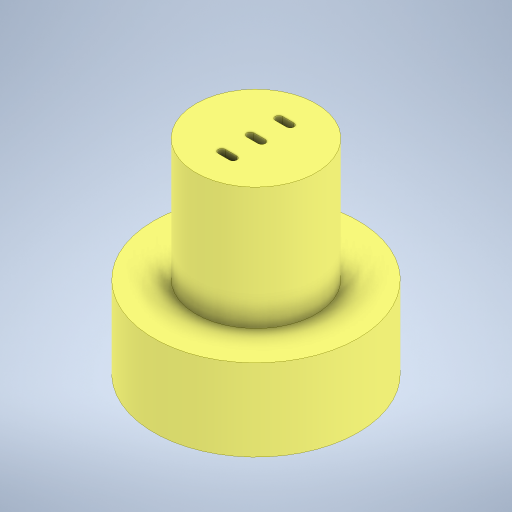
# Autodesk Inventor part: Kabelstopfen_Hinten_next try
Saved by Autodesk Inventor 2023 (Build 270158030, 158C)
## iProperties
Created: 2020-02-25
Part Number: Kabelstopfen_Hinten_next try
Material: Generic
Document SubType Name: Modeling
Designer: Julian
Density: 1 g/cm^3
Appearance: Default
Author: Julian
Autodesk Inventor part; units mm, degrees
ref_plane "YZ Plane" through (0, 0, 0) normal (1, 0, 0) x (0, 1, 0)
ref_plane "XZ Plane" through (0, 0, 0) normal (0, 1, 0) x (-1, 0, 0)
ref_plane "XY Plane" through (0, 0, 0) normal (0, 0, 1) x (1, 0, 0)
sketch "Sketch1" plane through (0, 0, 0) normal (0, 1, 0) x (-1, 0, 0)
  circle A0 centre (0.2, 0) radius 7.35
  circle A1 centre (0.2, 0) radius 12.5
  line L0 (0.2, 0) -> (0.2, -3.5)
  line L1 (0.2, 0) -> (0.2, 3.5)
  line L2 (0.2, 3.5) -> (-0.5, 3.5)
  line L3 (-0.5, 3.5) -> (0.9, 3.5)
  line L4 (0.2, 0) -> (-0.5, 0)
  line L5 (-0.5, 0) -> (0.9, 0)
  line L6 (0.2, -3.5) -> (-0.5, -3.5)
  line L7 (-0.5, -3.5) -> (0.9, -3.5)
  circle A2 centre (-0.5, -3.5) radius 0.45
  circle A3 centre (0.9, -3.5) radius 0.45
  circle A4 centre (-0.5, 0) radius 0.45
  circle A5 centre (0.9, 0) radius 0.45
  circle A6 centre (-0.5, 3.5) radius 0.45
  circle A7 centre (0.9, 3.5) radius 0.45
  line L8 (0.9, -3.95) -> (-0.5, -3.95)
  line L9 (-0.5, -3.05) -> (0.9, -3.05)
  line L10 (0.9, -0.45) -> (-0.5, -0.45)
  line L11 (-0.5, 0.45) -> (0.9, 0.45)
  line L12 (-0.5, 3.05) -> (0.9, 3.05)
  line L13 (-0.5, 3.95) -> (0.9, 3.95)
  line L14 (1.35, 3.5) -> (1.35, -3.5)
  dimension "d0" = 14.7
  dimension "d1" = 25
  dimension "d14" = 3.5
  dimension "d15" = 3.5
  dimension "d16" = 0.7
  dimension "d17" = 1.4
  dimension "d18" = 0.7
  dimension "d19" = 1.4
  dimension "d20" = 0.7
  dimension "d21" = 1.4
  dimension "d22" = 0.9
  dimension "d23" = 0.9
  dimension "d24" = 0.9
  dimension "d25" = 0.9
  dimension "d26" = 0.9
  dimension "d27" = 0.9
  constraints: 30 end point, 14 point on circle, 8 centre point, 7 coincident, 6 tangent, 3 horizontal, 3 point on line, 2 parallel, 2 vertical, 1 perpendicular
  measures "d0" diameter of A0
  measures "d1" diameter of A1
  measures "d14" distance of L0.start L0.end
  measures "d15" distance of L0.start L1.end
  measures "d16" distance of L1.end L2.end
  measures "d17" distance of L2.end L3.end
  measures "d18" distance of L0.start L4.end
  measures "d19" distance of L4.end L5.end
  measures "d20" distance of L0.end L6.end
  measures "d21" distance of L6.end L7.end
  measures "d22" diameter of A2
  measures "d23" diameter of A3
  measures "d24" diameter of A4
  measures "d25" diameter of A5
  measures "d26" diameter of A6
  measures "d27" diameter of A7
extrude "Extrusion1" add sketch "Sketch1" along normal blind 15 contours A0 | L10 A5 L14 A3 L9 L0 | L1 L12 A7 L14 A5 L11
extrude "Extrusion2" add sketch "Sketch1" against normal blind 10 contours A0 | A1 | L10 A5 L14 A3 L9 L0 | L1 L12 A7 L14 A5 L11
body "Solid1"
